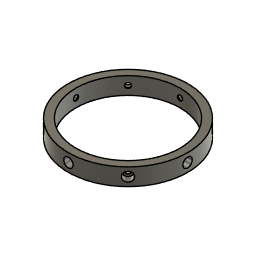
couplage_standard_femelle v11 (Autodesk Fusion 360 design; units mm, degrees)
Autodesk Fusion 360 part; units mm, degrees
sketch "Esquisse1" plane through (0, 0, 0) normal (0, 1, 0) x (1, 0, 0)
  circle A0 centre (0, 0) radius 35
  circle A1 centre (0, 0) radius 30
  dimension "d1" = 70
  dimension "d2" = 60
  constraint coincident A0.centre A1.centre
  constraint concentric A0 A1
  measures "d1" diameter of A0
  measures "d2" diameter of A1
extrude "Extrusion1" add sketch "Esquisse1" along normal mid plane 10
ref_plane "Plan de construction1" through (35, 0, 0) normal (1, 0, 0) x (0, 1, 0)
ref_plane "Plan de construction2" through (-35, 0, 0) normal (1, 0, 0) x (0, 1, 0)
ref_plane "Plan de construction3" through (0, 0, 35) normal (0, 0, 1) x (1, 0, 0)
ref_plane "Plan de construction4" through (0, 0, -35) normal (0, 0, 1) x (1, 0, 0)
sketch "Esquisse2" plane through (35, 0, 0) normal (1, 0, 0) x (0, 0, -1)
  circle A0 centre (0, 0) radius 1.5
  circle A1 centre (0, 0) radius 2.25
  dimension "d9" = 3
  dimension "d10" = 4.5
  constraint coincident A0.centre A1.centre
  constraint concentric A0 A1
  measures "d9" diameter of A0
  measures "d10" diameter of A1
extrude "Extrusion2" cut sketch "Esquisse2" against normal blind 70 contours A0
extrude "Extrusion3" cut sketch "Esquisse2" against normal blind 3
sketch "Esquisse3" plane through (-35, 0, 0) normal (1, 0, 0) x (0, 0, -1)
  circle A0 centre (0, 0) radius 2.25
  circle A1 centre (0, 0) radius 1.5
extrude "Extrusion4" cut sketch "Esquisse3" along normal blind 3
sketch "Esquisse4" plane through (0, 0, 35) normal (0, 0, 1) x (1, 0, 0)
  circle A0 centre (0, 0) radius 1.5
  circle A1 centre (0, 0) radius 2.25
  dimension "d17" = 3
  dimension "d18" = 4.5
  constraint coincident A0.centre A1.centre
  measures "d17" diameter of A0
  measures "d18" diameter of A1
extrude "Extrusion5" cut sketch "Esquisse4" against normal blind 70 contours A0
extrude "Extrusion6" cut sketch "Esquisse4" against normal blind 3
sketch "Esquisse5" plane through (0, 0, -35) normal (0, 0, 1) x (1, 0, 0)
  circle A0 centre (0, 0) radius 1.5
  circle A1 centre (0, 0) radius 2.25
extrude "Extrusion7" cut sketch "Esquisse5" along normal blind 3
move_body "Déplacer1" bodies 1 to x (0.707107, 0, 0.707107) y (0, 1, 0) z (-0.707107, 0, 0.707107) at (0, 0, 0)
ref_plane "Plan de construction5" through (35, 0, 0) normal (1, 0, 0) x (0, 1, 0)
ref_plane "Plan de construction6" through (-35, 0, 0) normal (1, 0, 0) x (0, 1, 0)
ref_plane "Plan de construction7" through (0, 0, 35) normal (0, 0, 1) x (1, 0, 0)
ref_plane "Plan de construction8" through (0, 0, -35) normal (0, 0, 1) x (1, 0, 0)
extrude "Extrusion8" cut sketch "Esquisse4" against normal blind 70 contours A0
extrude "Extrusion9" cut sketch "Esquisse4" against normal blind 3
sketch "Esquisse6" plane through (0, 0, -35) normal (0, 0, 1) x (1, 0, 0)
  circle A0 centre (0, 0) radius 2.25
  circle A1 centre (0, 0) radius 1.5
extrude "Extrusion10" cut sketch "Esquisse6" along normal blind 3
sketch "Esquisse7" plane through (-35, 0, 0) normal (1, 0, 0) x (0, 0, -1)
  circle A0 centre (0, 0) radius 1.5
  circle A1 centre (0, 0) radius 2.25
  dimension "d35" = 3
  dimension "d36" = 4.5
  constraint coincident A0.centre A1.centre
  measures "d35" diameter of A0
  measures "d36" diameter of A1
extrude "Extrusion11" cut sketch "Esquisse7" along normal blind 70 contours A0
extrude "Extrusion12" cut sketch "Esquisse7" along normal blind 3
sketch "Esquisse8" plane through (35, 0, 0) normal (1, 0, 0) x (0, 0, -1)
  circle A0 centre (0, 0) radius 2.25
  circle A1 centre (0, 0) radius 1.5
extrude "Extrusion13" cut sketch "Esquisse8" against normal blind 3
move_face "DécalerLesFaces1" offset -0.5 8 faces at (23.3345, 2.25, 23.3345) (33, 2.25, 0) (23.3345, 2.25, -23.3345) (0, 2.25, -33) (-23.3345, 2.25, -23.3345) (-33, 2.25, 0) (-23.3345, 2.25, 23.3345) (0, 2.25, 33)
extrude "Extrusion14" cut 1 faces at (32, -0.2111, -2.3175) along direction (-1, 0, 0) blind 1
extrude "Extrusion15" cut 1 faces at (24.2661, -0.2111, -20.9887) along direction (-0.707107, 0, 0.707107) blind 1
extrude "Extrusion16" cut 1 faces at (2.3231, -0.1366, -32) along direction (0, 0, 1) blind 1
extrude "Extrusion17" cut 1 faces at (-20.9847, -0.1366, -24.2701) along direction (0.707107, 0, 0.707107) blind 1
extrude "Extrusion18" cut 1 faces at (-32, -0.2111, -2.3175) along direction (1, 0, 0) blind 1
extrude "Extrusion19" cut 1 faces at (-20.9887, -0.2111, 24.2661) along direction (0.707107, 0, -0.707107) blind 1
extrude "Extrusion20" cut 1 faces at (2.3231, -0.1366, 32) along direction (0, 0, -1) blind 1
extrude "Extrusion21" cut 1 faces at (24.2701, -0.1366, 20.9847) along direction (-0.707107, 0, -0.707107) blind 1
move_face "DécalerLesFaces2" offset -0.5 1 faces at (-5.7003, -0.0323, 29.4535)
